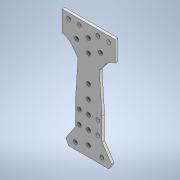
# Autodesk Inventor part: body_bone_3
Saved by Autodesk Inventor 2020 (Build 240168000, 168)
## iProperties
Created: 2019-05-16
Part Number: body_bone_3
Material: Generic
Document SubType Name: Modeling
Designer: psrob
Density: 1 g/cm^3
Appearance: Default
Author: psrob
Autodesk Inventor part; units mm, degrees
ref_plane "YZ Plane" through (0, 0, 0) normal (1, 0, 0) x (0, 1, 0)
ref_plane "XZ Plane" through (0, 0, 0) normal (0, 1, 0) x (-1, 0, 0)
ref_plane "XY Plane" through (0, 0, 0) normal (0, 0, 1) x (1, 0, 0)
sketch "Sketch1" plane through (0, 0, 0) normal (0, 0, 1) x (1, 0, 0)
  circle A0 centre (-34, 4) radius 1.5 projected
  circle A1 centre (-30, 13) radius 1.5 projected
  circle A2 centre (-27, 4) radius 1.5 projected
  line L0 (-30, 23) -> (-30, 40) projected
  line L1 (-40, 8) -> (-30, 23) projected
  line L2 (-40, 0) -> (-40, 8) projected
  line L3 (-40, 0) -> (-20, 0) projected
  line L4 (-20, 0) -> (-20, 40) projected
  line L5 (-20, 40) -> (-30, 40) projected
  circle A3 centre (-6, 4) radius 1.5 projected
  circle A4 centre (-10, 13) radius 1.5 projected
  circle A5 centre (-13, 4) radius 1.5 projected
  line L6 (-10, 23) -> (-10, 40) projected
  line L7 (-20, 40) -> (-10, 40) projected
  line L8 (-20, 0) -> (-20, 40) projected
  line L9 (0, 0) -> (-20, 0) projected
  line L10 (0, 0) -> (0, 8) projected
  line L11 (0, 8) -> (-10, 23) projected
  line L12 (0, 8) -> (-40, 8) projected
  circle A6 centre (-29, 80.8834) radius 1.5 projected
  circle A7 centre (-27, 90.8834) radius 1.5 projected
  circle A8 centre (-35, 90.8834) radius 1.5 projected
  line L13 (-40, 79.501) -> (-40, 94.8834) projected
  arc A9 (-32.05, 74.2834) -> (-40, 79.501) centre (-43.25, 65.8834) ccw projected
  line L14 (-28.0217, 68.9123) -> (-32.05, 74.2834) projected
  line L15 (-20, 68.9123) -> (-28.0217, 68.9123) projected
  line L16 (-20, 94.8834) -> (-20, 68.9123) projected
  line L17 (-40, 94.8834) -> (-20, 94.8834) projected
  circle A10 centre (-11, 80.8834) radius 1.5 projected
  circle A11 centre (-13, 90.8834) radius 1.5 projected
  circle A12 centre (-5, 90.8834) radius 1.5 projected
  line L18 (0, 79.501) -> (0, 94.8834) projected
  line L19 (0, 94.8834) -> (-20, 94.8834) projected
  line L20 (-20, 94.8834) -> (-20, 68.9123) projected
  line L21 (-20, 68.9123) -> (-11.9783, 68.9123) projected
  line L22 (-11.9783, 68.9123) -> (-7.95, 74.2834) projected
  arc A13 (0, 79.501) -> (-7.95, 74.2834) centre (3.25, 65.8834) ccw projected
  line L23 (-10, 40) -> (-11.9783, 68.9123)
  line L24 (-28.0217, 68.9123) -> (-30, 40)
  constraints: 4 end point
extrude "Extrusion1" add sketch "Sketch1" along normal blind 2 contours L0 L5 L4 L12 L1 | L24 L15 L21 L23 L7 L5 | L7 L6 L11 L12 L4 | L14 A9 L13 L17 L16 L15 | L16 L19 L18 A13 L22 L21
chamfer "Chamfer1" distance 5 angle 45 2 edges at (-40, 8, 1) (0, 8, 1)
sketch "Sketch2" plane through (0, 0, 2) normal (0, 0, 1) x (1, 0, 0)
  circle A0 centre (-27, 35.8834) radius 1.5 projected
  circle A1 centre (-13, 35.8834) radius 1.5 projected
  circle A2 centre (-13, 25.8834) radius 1.5 projected
  circle A3 centre (-27, 25.8834) radius 1.5 projected
  circle A4 centre (-20, 75.8834) radius 1.5 projected
  circle A5 centre (-20, 25.8834) radius 1.5 projected
  circle A6 centre (-20, 15.8834) radius 1.5 projected
  circle A7 centre (-20, 35.8834) radius 1.5 projected
  circle A8 centre (-20, 85.8834) radius 1.5 projected
  line L0 (-5, 8) -> (-2.7735, 12.1603) projected
  line L1 (-5, 8) -> (-35, 8) projected
  line L2 (-37.2265, 12.1603) -> (-35, 8) projected
  line L3 (-37.2265, 12.1603) -> (-30, 23) projected
  line L4 (-30, 23) -> (-30, 40) projected
  line L5 (-30, 40) -> (-26, 40) projected
  arc A9 (-26, 40) -> (-23, 43) centre (-26, 43) ccw projected
  line L6 (-23, 43) -> (-23, 65.9123) projected
  arc A10 (-23, 65.9123) -> (-26, 68.9123) centre (-26, 65.9123) ccw projected
  line L7 (-26, 68.9123) -> (-28.0217, 68.9123) projected
  line L8 (-28.0217, 68.9123) -> (-32.05, 74.2834) projected
  arc A11 (-32.05, 74.2834) -> (-40, 79.501) centre (-43.25, 65.8834) ccw projected
  line L9 (-40, 79.501) -> (-40, 94.8834) projected
  line L10 (-40, 94.8834) -> (0, 94.8834) projected
  line L11 (0, 94.8834) -> (0, 79.501) projected
  arc A12 (0, 79.501) -> (-7.95, 74.2834) centre (3.25, 65.8834) ccw projected
  line L12 (-7.95, 74.2834) -> (-11.9783, 68.9123) projected
  line L13 (-11.9783, 68.9123) -> (-14, 68.9123) projected
  arc A13 (-14, 68.9123) -> (-17, 65.9123) centre (-14, 65.9123) ccw projected
  line L14 (-17, 65.9123) -> (-17, 43) projected
  arc A14 (-17, 43) -> (-14, 40) centre (-14, 43) ccw projected
  line L15 (-14, 40) -> (-10, 40) projected
  line L16 (-10, 40) -> (-10, 23) projected
  line L17 (-10, 23) -> (-2.7735, 12.1603) projected
  circle A15 centre (-30, 13) radius 1.5 projected
  circle A16 centre (-27, 90.8834) radius 1.5 projected
  circle A17 centre (-29, 80.8834) radius 1.5 projected
  circle A18 centre (-35, 90.8834) radius 1.5 projected
  circle A19 centre (-11, 80.8834) radius 1.5 projected
  circle A20 centre (-13, 90.8834) radius 1.5 projected
  circle A21 centre (-5, 90.8834) radius 1.5 projected
  circle A22 centre (-10, 13) radius 1.5 projected
  point P0 (0, 0)
extrude "Extrusion2" cut sketch "Sketch2" against normal blind 10 contours A0 | A1 | A2 | A3 | A4 | A5 | A6 | A7 | A8
sketch "Sketch3" plane through (0, 0, 2) normal (0, 0, 1) x (1, 0, 0)
  circle A0 centre (-13, 35.8834) radius 1.5 projected
  circle A1 centre (-20, 35.8834) radius 1.5 projected
  circle A2 centre (-27, 35.8834) radius 1.5 projected
  circle A3 centre (-13, 25.8834) radius 1.5 projected
  circle A4 centre (-20, 75.8834) radius 1.5 projected
  circle A5 centre (-20, 25.8834) radius 1.5 projected
  circle A6 centre (-27, 25.8834) radius 1.5 projected
  circle A7 centre (-20, 15.8834) radius 1.5 projected
  circle A8 centre (-20, 85.8834) radius 1.5 projected
  line L0 (-2.7735, 12.1603) -> (-5, 8) projected
  line L1 (-2.7735, 12.1603) -> (-10, 23) projected
  line L2 (-10, 23) -> (-10, 40) projected
  line L3 (-10, 40) -> (-11.9783, 68.9123) projected
  line L4 (-11.9783, 68.9123) -> (-7.95, 74.2834) projected
  arc A9 (0, 79.501) -> (-7.95, 74.2834) centre (3.25, 65.8834) ccw projected
  line L5 (0, 79.501) -> (0, 94.8834) projected
  line L6 (0, 94.8834) -> (-40, 94.8834) projected
  line L7 (-40, 94.8834) -> (-40, 79.501) projected
  arc A10 (-32.05, 74.2834) -> (-40, 79.501) centre (-43.25, 65.8834) ccw projected
  line L8 (-32.05, 74.2834) -> (-28.0217, 68.9123) projected
  line L9 (-28.0217, 68.9123) -> (-30, 40) projected
  line L10 (-30, 40) -> (-30, 23) projected
  line L11 (-30, 23) -> (-37.2265, 12.1603) projected
  line L12 (-35, 8) -> (-37.2265, 12.1603) projected
  line L13 (-35, 8) -> (-5, 8) projected
  circle A11 centre (-13, 90.8834) radius 1.5 projected
  circle A12 centre (-11, 80.8834) radius 1.5 projected
  circle A13 centre (-5, 90.8834) radius 1.5 projected
  circle A14 centre (-29, 80.8834) radius 1.5 projected
  circle A15 centre (-27, 90.8834) radius 1.5 projected
  circle A16 centre (-35, 90.8834) radius 1.5 projected
  circle A17 centre (-30, 13) radius 1.5 projected
  circle A18 centre (-10, 13) radius 1.5 projected
  circle A19 centre (-20, 75.8834) radius 1.5 projected
  line L14 (-20, 75.8834) -> (-20, 55.8834)
  line L15 (-20, 55.8834) -> (-20, 45.8834)
  circle A20 centre (-20, 55.8834) radius 1.5
  circle A21 centre (-20, 45.8834) radius 1.5
  point P0 (0, 0)
  dimension "d7" = 20
  dimension "d8" = 10
  dimension "d9" = 3
  dimension "d10" = 3
  constraints: 4 end point, 2 centre point, 2 coincident, 1 point on line, 1 vertical
  measures "d7" distance of L14.start L14.end
  measures "d8" distance of L14.end L15.end
  measures "d9" diameter of A20
  measures "d10" diameter of A21
extrude "Extrusion3" cut sketch "Sketch3" against normal blind 10 contours A20 L15 L14 | L14 L15 A20 | A21
body "Solid1"
